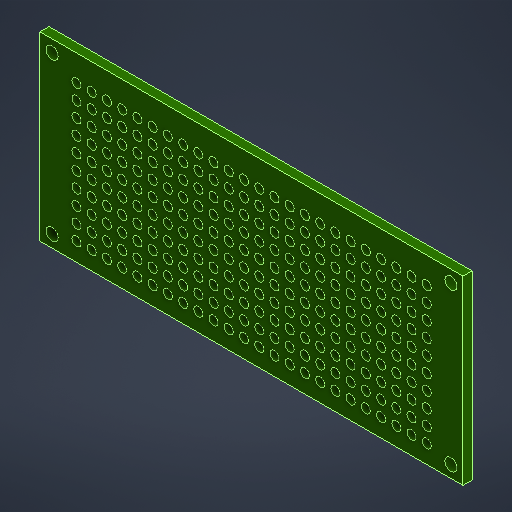
# Autodesk Inventor part: P_PCB_40x60
Saved by Autodesk Inventor 2026 (Build 300175000, 175)
## iProperties
Created: 2025-09-06
Part Number: P_PCB_40x60
Material: Generisch
Document SubType Name: Modeling
Designer: FAL
Density: 1 g/cm^3
Appearance: Vorgabe
Author: FAL
Autodesk Inventor part; units mm, degrees
ref_plane "YZ Plane" through (0, 0, 0) normal (1, 0, 0) x (0, 1, 0)
ref_plane "XZ Plane" through (0, 0, 0) normal (0, 1, 0) x (-1, 0, 0)
ref_plane "XY Plane" through (0, 0, 0) normal (0, 0, 1) x (1, 0, 0)
sketch "Skizze1" plane through (0, 0, 0) normal (0, 1, 0) x (-1, 0, 0)
  line L0 (-35, 15) -> (35, 15)
  line L1 (35, 15) -> (35, -15)
  line L2 (35, -15) -> (-35, -15)
  line L3 (-35, -15) -> (-35, 15)
  line L4 (-35, 15) -> (35, -15) construction
  line L5 (35, 15) -> (-35, -15) construction
  point P0 (0, 0)
  dimension "d0" = 30
  dimension "d1" = 70
  constraints: 12 end point, 2 midpoint, 2 parallel, 1 horizontal, 1 perpendicular
  measures "d0" distance between parallel lines of L2 L0
  measures "d1" distance of L1.end L2.end
extrude "Extrusion1" add sketch "Skizze1" along normal blind 1.5
sketch "Skizze2" plane through (0, 0, 0) normal (0, 1, 0) x (-1, 0, 0)
  line L0 (33, 13) -> (-33, 13) construction
  line L1 (-33, 13) -> (-33, -13) construction
  line L2 (-33, -13) -> (33, -13) construction
  line L3 (33, -13) -> (33, 13) construction
  line L4 (33, 13) -> (-33, -13) construction
  line L5 (-33, 13) -> (33, -13) construction
  circle A0 centre (-33, -13) radius 1
  circle A1 centre (-33, 13) radius 1
  circle A2 centre (33, 13) radius 1
  circle A3 centre (33, -13) radius 1
  point P0 (0, 0)
  dimension "d4" = 26
  dimension "d5" = 66
  dimension "d6" = 2
  constraints: 12 end point, 4 centre point, 4 coincident, 3 equal radius, 2 midpoint, 2 parallel, 1 horizontal, 1 perpendicular
  measures "d4" distance of L2.end L0.start
  measures "d5" distance of L1.end L2.end
  measures "d6" diameter of A0
extrude "Extrusion2" cut sketch "Skizze2" along normal blind 6
sketch "Skizze3" plane through (0, 0, 0) normal (0, 1, 0) x (-1, 0, 0)
  circle A0 centre (-29, -12) radius 0.75
  line L0 (-35, -15) -> (35, -15) projected
  line L1 (-35, 15) -> (-35, -15) projected
  circle A1 centre (-26.48, -12) radius 0.75
  circle A2 centre (-23.96, -12) radius 0.75
  circle A3 centre (-21.44, -12) radius 0.75
  circle A4 centre (-18.92, -12) radius 0.75
  circle A5 centre (-16.4, -12) radius 0.75
  circle A6 centre (-13.88, -12) radius 0.75
  circle A7 centre (-11.36, -12) radius 0.75
  circle A8 centre (-8.84, -12) radius 0.75
  circle A9 centre (-6.32, -12) radius 0.75
  circle A10 centre (-3.8, -12) radius 0.75
  circle A11 centre (-1.28, -12) radius 0.75
  circle A12 centre (1.24, -12) radius 0.75
  circle A13 centre (3.76, -12) radius 0.75
  circle A14 centre (6.28, -12) radius 0.75
  circle A15 centre (8.8, -12) radius 0.75
  circle A16 centre (11.32, -12) radius 0.75
  circle A17 centre (13.84, -12) radius 0.75
  circle A18 centre (16.36, -12) radius 0.75
  circle A19 centre (18.88, -12) radius 0.75
  circle A20 centre (-29, -9.48) radius 0.75
  circle A21 centre (-26.48, -9.48) radius 0.75
  circle A22 centre (-23.96, -9.48) radius 0.75
  circle A23 centre (-21.44, -9.48) radius 0.75
  circle A24 centre (-18.92, -9.48) radius 0.75
  circle A25 centre (-16.4, -9.48) radius 0.75
  circle A26 centre (-13.88, -9.48) radius 0.75
  circle A27 centre (-11.36, -9.48) radius 0.75
  circle A28 centre (-8.84, -9.48) radius 0.75
  circle A29 centre (-6.32, -9.48) radius 0.75
  circle A30 centre (-3.8, -9.48) radius 0.75
  circle A31 centre (-1.28, -9.48) radius 0.75
  circle A32 centre (1.24, -9.48) radius 0.75
  circle A33 centre (3.76, -9.48) radius 0.75
  circle A34 centre (6.28, -9.48) radius 0.75
  circle A35 centre (8.8, -9.48) radius 0.75
  circle A36 centre (11.32, -9.48) radius 0.75
  circle A37 centre (13.84, -9.48) radius 0.75
  circle A38 centre (16.36, -9.48) radius 0.75
  circle A39 centre (18.88, -9.48) radius 0.75
  circle A40 centre (-29, -6.96) radius 0.75
  circle A41 centre (-26.48, -6.96) radius 0.75
  circle A42 centre (-23.96, -6.96) radius 0.75
  circle A43 centre (-21.44, -6.96) radius 0.75
  circle A44 centre (-18.92, -6.96) radius 0.75
  circle A45 centre (-16.4, -6.96) radius 0.75
  circle A46 centre (-13.88, -6.96) radius 0.75
  circle A47 centre (-11.36, -6.96) radius 0.75
  circle A48 centre (-8.84, -6.96) radius 0.75
  circle A49 centre (-6.32, -6.96) radius 0.75
  circle A50 centre (-3.8, -6.96) radius 0.75
  circle A51 centre (-1.28, -6.96) radius 0.75
  circle A52 centre (1.24, -6.96) radius 0.75
  circle A53 centre (3.76, -6.96) radius 0.75
  circle A54 centre (6.28, -6.96) radius 0.75
  circle A55 centre (8.8, -6.96) radius 0.75
  circle A56 centre (11.32, -6.96) radius 0.75
  circle A57 centre (13.84, -6.96) radius 0.75
  circle A58 centre (16.36, -6.96) radius 0.75
  circle A59 centre (18.88, -6.96) radius 0.75
  circle A60 centre (-29, -4.44) radius 0.75
  circle A61 centre (-26.48, -4.44) radius 0.75
  circle A62 centre (-23.96, -4.44) radius 0.75
  circle A63 centre (-21.44, -4.44) radius 0.75
  circle A64 centre (-18.92, -4.44) radius 0.75
  circle A65 centre (-16.4, -4.44) radius 0.75
  circle A66 centre (-13.88, -4.44) radius 0.75
  circle A67 centre (-11.36, -4.44) radius 0.75
  circle A68 centre (-8.84, -4.44) radius 0.75
  circle A69 centre (-6.32, -4.44) radius 0.75
  circle A70 centre (-3.8, -4.44) radius 0.75
  circle A71 centre (-1.28, -4.44) radius 0.75
  circle A72 centre (1.24, -4.44) radius 0.75
  circle A73 centre (3.76, -4.44) radius 0.75
  circle A74 centre (6.28, -4.44) radius 0.75
  circle A75 centre (8.8, -4.44) radius 0.75
  circle A76 centre (11.32, -4.44) radius 0.75
  circle A77 centre (13.84, -4.44) radius 0.75
  circle A78 centre (16.36, -4.44) radius 0.75
  circle A79 centre (18.88, -4.44) radius 0.75
  circle A80 centre (-29, -1.92) radius 0.75
  circle A81 centre (-26.48, -1.92) radius 0.75
  circle A82 centre (-23.96, -1.92) radius 0.75
  circle A83 centre (-21.44, -1.92) radius 0.75
  circle A84 centre (-18.92, -1.92) radius 0.75
  circle A85 centre (-16.4, -1.92) radius 0.75
  circle A86 centre (-13.88, -1.92) radius 0.75
  circle A87 centre (-11.36, -1.92) radius 0.75
  circle A88 centre (-8.84, -1.92) radius 0.75
  circle A89 centre (-6.32, -1.92) radius 0.75
  circle A90 centre (-3.8, -1.92) radius 0.75
  circle A91 centre (-1.28, -1.92) radius 0.75
  circle A92 centre (1.24, -1.92) radius 0.75
  circle A93 centre (3.76, -1.92) radius 0.75
  circle A94 centre (6.28, -1.92) radius 0.75
  circle A95 centre (8.8, -1.92) radius 0.75
  circle A96 centre (11.32, -1.92) radius 0.75
  circle A97 centre (13.84, -1.92) radius 0.75
  circle A98 centre (16.36, -1.92) radius 0.75
  circle A99 centre (18.88, -1.92) radius 0.75
  circle A100 centre (-29, 0.6) radius 0.75
  circle A101 centre (-26.48, 0.6) radius 0.75
  circle A102 centre (-23.96, 0.6) radius 0.75
  circle A103 centre (-21.44, 0.6) radius 0.75
  circle A104 centre (-18.92, 0.6) radius 0.75
  circle A105 centre (-16.4, 0.6) radius 0.75
  circle A106 centre (-13.88, 0.6) radius 0.75
  circle A107 centre (-11.36, 0.6) radius 0.75
  circle A108 centre (-8.84, 0.6) radius 0.75
  circle A109 centre (-6.32, 0.6) radius 0.75
  circle A110 centre (-3.8, 0.6) radius 0.75
  circle A111 centre (-1.28, 0.6) radius 0.75
  circle A112 centre (1.24, 0.6) radius 0.75
  circle A113 centre (3.76, 0.6) radius 0.75
  circle A114 centre (6.28, 0.6) radius 0.75
  circle A115 centre (8.8, 0.6) radius 0.75
  circle A116 centre (11.32, 0.6) radius 0.75
  circle A117 centre (13.84, 0.6) radius 0.75
  circle A118 centre (16.36, 0.6) radius 0.75
  circle A119 centre (18.88, 0.6) radius 0.75
  circle A120 centre (-29, 3.12) radius 0.75
  circle A121 centre (-26.48, 3.12) radius 0.75
  circle A122 centre (-23.96, 3.12) radius 0.75
  circle A123 centre (-21.44, 3.12) radius 0.75
  circle A124 centre (-18.92, 3.12) radius 0.75
  circle A125 centre (-16.4, 3.12) radius 0.75
  circle A126 centre (-13.88, 3.12) radius 0.75
  circle A127 centre (-11.36, 3.12) radius 0.75
  circle A128 centre (-8.84, 3.12) radius 0.75
  circle A129 centre (-6.32, 3.12) radius 0.75
  circle A130 centre (-3.8, 3.12) radius 0.75
  circle A131 centre (-1.28, 3.12) radius 0.75
  circle A132 centre (1.24, 3.12) radius 0.75
  circle A133 centre (3.76, 3.12) radius 0.75
  circle A134 centre (6.28, 3.12) radius 0.75
  circle A135 centre (8.8, 3.12) radius 0.75
  circle A136 centre (11.32, 3.12) radius 0.75
  circle A137 centre (13.84, 3.12) radius 0.75
  circle A138 centre (16.36, 3.12) radius 0.75
  circle A139 centre (18.88, 3.12) radius 0.75
  circle A140 centre (-29, 5.64) radius 0.75
  circle A141 centre (-26.48, 5.64) radius 0.75
  circle A142 centre (-23.96, 5.64) radius 0.75
  circle A143 centre (-21.44, 5.64) radius 0.75
  circle A144 centre (-18.92, 5.64) radius 0.75
  circle A145 centre (-16.4, 5.64) radius 0.75
  circle A146 centre (-13.88, 5.64) radius 0.75
  circle A147 centre (-11.36, 5.64) radius 0.75
  circle A148 centre (-8.84, 5.64) radius 0.75
  circle A149 centre (-6.32, 5.64) radius 0.75
  circle A150 centre (-3.8, 5.64) radius 0.75
  circle A151 centre (-1.28, 5.64) radius 0.75
  circle A152 centre (1.24, 5.64) radius 0.75
  circle A153 centre (3.76, 5.64) radius 0.75
  circle A154 centre (6.28, 5.64) radius 0.75
  circle A155 centre (8.8, 5.64) radius 0.75
  circle A156 centre (11.32, 5.64) radius 0.75
  circle A157 centre (13.84, 5.64) radius 0.75
  circle A158 centre (16.36, 5.64) radius 0.75
  circle A159 centre (18.88, 5.64) radius 0.75
  circle A160 centre (-29, 8.16) radius 0.75
  circle A161 centre (-26.48, 8.16) radius 0.75
  circle A162 centre (-23.96, 8.16) radius 0.75
  circle A163 centre (-21.44, 8.16) radius 0.75
  circle A164 centre (-18.92, 8.16) radius 0.75
  circle A165 centre (-16.4, 8.16) radius 0.75
  circle A166 centre (-13.88, 8.16) radius 0.75
  circle A167 centre (-11.36, 8.16) radius 0.75
  circle A168 centre (-8.84, 8.16) radius 0.75
  circle A169 centre (-6.32, 8.16) radius 0.75
  circle A170 centre (-3.8, 8.16) radius 0.75
  circle A171 centre (-1.28, 8.16) radius 0.75
  circle A172 centre (1.24, 8.16) radius 0.75
  circle A173 centre (3.76, 8.16) radius 0.75
  circle A174 centre (6.28, 8.16) radius 0.75
  circle A175 centre (8.8, 8.16) radius 0.75
  circle A176 centre (11.32, 8.16) radius 0.75
  circle A177 centre (13.84, 8.16) radius 0.75
  circle A178 centre (16.36, 8.16) radius 0.75
  circle A179 centre (18.88, 8.16) radius 0.75
  circle A180 centre (21.4, -12) radius 0.75
  circle A181 centre (21.4, -9.48) radius 0.75
  circle A182 centre (21.4, -6.96) radius 0.75
  circle A183 centre (21.4, -4.44) radius 0.75
  circle A184 centre (21.4, -1.92) radius 0.75
  circle A185 centre (21.4, 0.6) radius 0.75
  circle A186 centre (21.4, 3.12) radius 0.75
  circle A187 centre (21.4, 5.64) radius 0.75
  circle A188 centre (21.4, 8.16) radius 0.75
  circle A189 centre (23.92, -12) radius 0.75
  circle A190 centre (23.92, -9.48) radius 0.75
  circle A191 centre (23.92, -6.96) radius 0.75
  circle A192 centre (23.92, -4.44) radius 0.75
  circle A193 centre (23.92, -1.92) radius 0.75
  circle A194 centre (23.92, 0.6) radius 0.75
  circle A195 centre (23.92, 3.12) radius 0.75
  circle A196 centre (23.92, 5.64) radius 0.75
  circle A197 centre (23.92, 8.16) radius 0.75
  circle A198 centre (26.44, -12) radius 0.75
  circle A199 centre (26.44, -9.48) radius 0.75
  circle A200 centre (26.44, -6.96) radius 0.75
  circle A201 centre (26.44, -4.44) radius 0.75
  circle A202 centre (26.44, -1.92) radius 0.75
  circle A203 centre (26.44, 0.6) radius 0.75
  circle A204 centre (26.44, 3.12) radius 0.75
  circle A205 centre (26.44, 5.64) radius 0.75
  circle A206 centre (26.44, 8.16) radius 0.75
  circle A207 centre (28.96, -12) radius 0.75
  circle A208 centre (28.96, -9.48) radius 0.75
  circle A209 centre (28.96, -6.96) radius 0.75
  circle A210 centre (28.96, -4.44) radius 0.75
  circle A211 centre (28.96, -1.92) radius 0.75
  circle A212 centre (28.96, 0.6) radius 0.75
  circle A213 centre (28.96, 3.12) radius 0.75
  circle A214 centre (28.96, 5.64) radius 0.75
  circle A215 centre (28.96, 8.16) radius 0.75
  circle A216 centre (-29, 10.68) radius 0.75
  circle A217 centre (-26.48, 10.68) radius 0.75
  circle A218 centre (-23.96, 10.68) radius 0.75
  circle A219 centre (-21.44, 10.68) radius 0.75
  circle A220 centre (-18.92, 10.68) radius 0.75
  circle A221 centre (-16.4, 10.68) radius 0.75
  circle A222 centre (-13.88, 10.68) radius 0.75
  circle A223 centre (-11.36, 10.68) radius 0.75
  circle A224 centre (-8.84, 10.68) radius 0.75
  circle A225 centre (-6.32, 10.68) radius 0.75
  circle A226 centre (-3.8, 10.68) radius 0.75
  circle A227 centre (-1.28, 10.68) radius 0.75
  circle A228 centre (1.24, 10.68) radius 0.75
  circle A229 centre (3.76, 10.68) radius 0.75
  circle A230 centre (6.28, 10.68) radius 0.75
  circle A231 centre (8.8, 10.68) radius 0.75
  circle A232 centre (11.32, 10.68) radius 0.75
  circle A233 centre (13.84, 10.68) radius 0.75
  circle A234 centre (16.36, 10.68) radius 0.75
  circle A235 centre (18.88, 10.68) radius 0.75
  circle A236 centre (21.4, 10.68) radius 0.75
  circle A237 centre (23.92, 10.68) radius 0.75
  circle A238 centre (26.44, 10.68) radius 0.75
  circle A239 centre (28.96, 10.68) radius 0.75
  point P0 (0, 0)
  dimension "d9" = 1.5
  dimension "d10" = 3
  dimension "d11" = 6
  dimension "d14" = 2.52
  dimension "d17" = 2.52
  constraints: 240 centre point, 1 horizontal, 1 vertical, 478 other
  measures "d9" diameter of A0
  measures "d10" distance from line of L0 A0.centre
  measures "d11" distance from line of L1 A0.centre
  measures "d14" distance of A0.centre A1.centre
  measures "d17" distance of A0.centre A20.centre
extrude "Extrusion4" cut sketch "Skizze3" along normal blind 10
